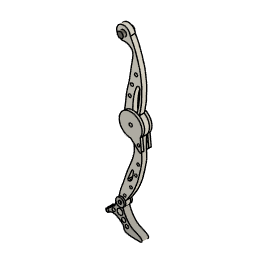
3R Planner Leg (Autodesk Fusion 360 design; units mm, degrees)
Autodesk Fusion 360 part; units mm, degrees
note: some values were not read from the file. Chosen so that the rebuilt part matches the saved one: which face or edge a step refers to. Set by a fixed rule: which sketch regions a step uses.
sketch "Sketch Thigh" plane through (0, 0, 0) normal (0, 1, 0) x (1, 0, 0)
  circle A0 centre (-35.2013, -526.5286) radius 18
  circle A1 centre (-35.2013, -526.5286) radius 42
  circle A2 centre (23.3414, -77.3372) radius 10
  circle A3 centre (23.3414, -77.3372) radius 70
  spline S0 degree 5 poles (-36.4317, -484.5466) (-35.2037, -484.7809) (-32.7765, -485.1866) (-29.2218, -485.606) (-24.6544, -485.7869) (-19.2317, -485.3906) (-14.0932, -484.3977) (-9.2342, -482.86) (-4.6456, -480.8668) (-0.3151, -478.5474) (3.7633, -476.0289) (7.5794, -473.3959) (11.0975, -470.6537) (14.2448, -467.6799) (16.9324, -464.2887) (19.0817, -460.3121) (20.6487, -455.6738) (21.6499, -450.4697) (22.1462, -444.906) (22.2249, -439.2304) (21.9831, -433.6701) (21.5089, -428.3588) (20.8685, -423.2931) (20.1126, -418.3916) (19.2797, -413.5384) (18.4002, -408.6286) (17.5013, -403.6235) (16.6061, -398.5439) (15.7315, -393.4337) (14.8853, -388.3343) (14.0639, -383.2529) (13.2508, -378.1395) (12.4244, -372.9172) (11.5642, -367.5091) (10.6578, -361.8637) (9.7092, -355.9869) (8.7399, -349.9497) (7.778, -343.8514) (6.85, -337.7941) (5.972, -331.8527) (5.1403, -326.0462) (4.323, -320.3093) (3.4714, -314.5275) (2.5311, -308.5697) (1.4536, -302.3234) (0.2063, -295.725) (-1.2135, -288.8021) (-2.7809, -281.6615) (-4.4528, -274.4499) (-6.1756, -267.3234) (-7.8935, -260.4128) (-9.5563, -253.7929) (-11.1279, -247.4427) (-12.5916, -241.2351) (-13.9437, -234.9891) (-15.1909, -228.5075) (-16.3452, -221.6232) (-17.4211, -214.2368) (-18.4302, -206.3689) (-19.3796, -198.1708) (-20.2738, -189.8721) (-21.1157, -181.7419) (-21.908, -174.0454) (-22.6546, -167.0005) (-23.3615, -160.7395) (-24.0388, -155.2553) (-24.7002, -150.407) (-25.3606, -145.9837) (-26.0341, -141.7521) (-26.7323, -137.512) (-27.4617, -133.1445) (-28.073, -129.5011) (-28.5476, -126.6757) (-28.8711, -124.7508) (-29.0347, -123.778) knots 0 0 0 0 0 0 0.01428571 0.02857143 0.04285714 0.05714286 0.07142857 0.08571429 0.1 0.11428571 0.12857143 0.14285714 0.15714286 0.17142857 0.18571429 0.2 0.21428571 0.22857143 0.24285714 0.25714286 0.27142857 0.28571429 0.3 0.31428571 0.32857143 0.34285714 0.35714286 0.37142857 0.38571429 0.4 0.41428571 0.42857143 0.44285714 0.45714286 0.47142857 0.48571429 0.5 0.51428571 0.52857143 0.54285714 0.55714286 0.57142857 0.58571429 0.6 0.61428571 0.62857143 0.64285714 0.65714286 0.67142857 0.68571429 0.7 0.71428571 0.72857143 0.74285714 0.75714286 0.77142857 0.78571429 0.8 0.81428571 0.82857143 0.84285714 0.85714286 0.87142857 0.88571429 0.9 0.91428571 0.92857143 0.94285714 0.95714286 0.97142857 0.98571429 1 1 1 1 1 1
  spline S1 degree 5 poles (6.5737, -530.8697) (7.0819, -529.9673) (8.0856, -528.1802) (9.5529, -525.5529) (11.4329, -522.1561) (13.6572, -518.0832) (15.7611, -514.1707) (17.7553, -510.3927) (19.6573, -506.7066) (21.4946, -503.0462) (23.3012, -499.3289) (25.1103, -495.4746) (26.9465, -491.4225) (28.8195, -487.1472) (30.7152, -482.6796) (32.5963, -478.1064) (34.4167, -473.5372) (36.1326, -469.0815) (37.7154, -464.8201) (39.1618, -460.7812) (40.5096, -456.9081) (41.8236, -453.0843) (43.175, -449.1724) (44.6223, -445.0502) (46.1931, -440.6451) (47.8612, -435.9764) (49.5592, -431.1398) (51.2018, -426.2744) (52.7052, -421.5361) (54.0089, -417.0681) (55.0953, -412.9726) (56.0117, -409.2816) (56.843, -405.9653) (57.681, -402.941) (58.5978, -400.0837) (59.6103, -397.2324) (60.6872, -394.2152) (61.7771, -390.8838) (62.8289, -387.1428) (63.8193, -382.9883) (64.7487, -378.4906) (65.6314, -373.763) (66.4863, -368.9347) (67.3285, -364.1236) (68.1587, -359.4042) (68.9603, -354.7957) (69.7099, -350.2839) (70.3847, -345.8343) (70.971, -341.4096) (71.472, -336.9843) (71.9171, -332.5629) (72.3503, -328.1702) (72.8161, -323.8408) (73.3463, -319.6081) (73.9477, -315.4945) (74.5851, -311.4985) (75.1935, -307.5983) (75.7011, -303.7607) (76.0491, -299.9491) (76.2129, -296.1312) (76.2219, -292.2868) (76.1379, -288.4024) (76.0325, -284.4647) (75.9672, -280.4559) (75.9671, -276.346) (76.0138, -272.0939) (76.0664, -267.6643) (76.0766, -263.0405) (76.0051, -258.2381) (75.8395, -253.3208) (75.6065, -248.4083) (75.3539, -243.6407) (75.136, -239.1482) (74.9971, -235.0179) (74.9579, -231.2653) (74.9959, -227.7929) (75.0547, -224.4212) (75.0665, -220.9505) (74.9679, -217.2076) (74.7222, -213.1105) (74.3246, -208.6794) (73.7907, -203.9948) (73.1489, -199.1682) (72.4317, -194.3094) (71.667, -189.4932) (70.8708, -184.7318) (70.0508, -180.0012) (69.2089, -175.2609) (68.3451, -170.4763) (67.4591, -165.6392) (66.5545, -160.7927) (65.6399, -156.0379) (64.7262, -151.5067) (63.8253, -147.3427) (62.9484, -143.6795) (62.1039, -140.6187) (61.4576, -138.6919) (60.9899, -137.548) (60.6857, -136.9191) (60.5355, -136.6381) knots 0 0 0 0 0 0 0.01052632 0.02105263 0.03157895 0.04210526 0.05263158 0.06315789 0.07368421 0.08421053 0.09473684 0.10526316 0.11578947 0.12631579 0.13684211 0.14736842 0.15789474 0.16842105 0.17894737 0.18947368 0.2 0.21052632 0.22105263 0.23157895 0.24210526 0.25263158 0.26315789 0.27368421 0.28421053 0.29473684 0.30526316 0.31578947 0.32631579 0.33684211 0.34736842 0.35789474 0.36842105 0.37894737 0.38947368 0.4 0.41052632 0.42105263 0.43157895 0.44210526 0.45263158 0.46315789 0.47368421 0.48421053 0.49473684 0.50526316 0.51578947 0.52631579 0.53684211 0.54736842 0.55789474 0.56842105 0.57894737 0.58947368 0.6 0.61052632 0.62105263 0.63157895 0.64210526 0.65263158 0.66315789 0.67368421 0.68421053 0.69473684 0.70526316 0.71578947 0.72631579 0.73684211 0.74736842 0.75789474 0.76842105 0.77894737 0.78947368 0.8 0.81052632 0.82105263 0.83157895 0.84210526 0.85263158 0.86315789 0.87368421 0.88421053 0.89473684 0.90526316 0.91578947 0.92631579 0.93684211 0.94736842 0.95789474 0.96842105 0.97894737 0.98947368 1 1 1 1 1 1
  circle A4 centre (55, -280) radius 9
  circle A5 centre (30, -120) radius 9
  spline S2 degree 5 poles (47.6191, -285.15) (46.8064, -283.5762) (45.2153, -280.4019) (42.9311, -275.5604) (40.0915, -268.9442) (36.8892, -260.4073) (34.038, -251.6146) (31.5388, -242.5934) (29.3866, -233.394) (27.5666, -224.0998) (26.0533, -214.8264) (24.8152, -205.7002) (23.8182, -196.8425) (23.0287, -188.3502) (22.4171, -180.2791) (21.9607, -172.6203) (21.6435, -165.3143) (21.4545, -158.2753) (21.3865, -151.4109) (21.4343, -144.6444) (21.5935, -137.9312) (21.8074, -132.585) (22.0156, -128.5856) (22.1756, -125.9238) (22.2609, -124.5941) knots 0 0 0 0 0 0 0.05 0.1 0.15 0.2 0.25 0.3 0.35 0.4 0.45 0.5 0.55 0.6 0.65 0.7 0.75 0.8 0.85 0.9 0.95 1 1 1 1 1 1
  spline S3 degree 5 poles (63.9903, -280.4171) (63.9954, -279.3418) (63.9944, -277.1207) (63.9589, -273.5771) (63.8437, -268.427) (63.5836, -261.2767) (63.2024, -253.4204) (62.6917, -244.885) (62.0399, -235.7314) (61.2328, -226.0534) (60.2567, -215.9694) (59.1004, -205.6177) (57.7586, -195.15) (56.2338, -184.7277) (54.5407, -174.5163) (52.7057, -164.6805) (50.7617, -155.3773) (48.7441, -146.749) (46.6866, -138.9154) (44.6174, -131.9666) (42.5545, -125.9502) (40.916, -121.8936) (39.695, -119.2752) (38.8845, -117.7173) (38.4801, -116.9853) knots 0 0 0 0 0 0 0.05 0.1 0.15 0.2 0.25 0.3 0.35 0.4 0.45 0.5 0.55 0.6 0.65 0.7 0.75 0.8 0.85 0.9 0.95 1 1 1 1 1 1
  circle A6 centre (41.2295, -343.8614) radius 9
  circle A7 centre (16.4257, -279.8469) radius 9
  circle A8 centre (3.0698, -214.2122) radius 9
  point P0 (-10, -483)
  point P1 (8, -473)
  point P2 (19, -460)
  point P3 (22, -435)
  point P4 (19, -412)
  point P5 (15, -389)
  point P6 (11, -364)
  point P7 (6, -332)
  point P8 (1, -300)
  point P9 (-9, -256)
  point P10 (-17, -217)
  point P11 (-23, -164)
  point P12 (-26, -142)
  point P13 (18.658, -508.6317)
  point P14 (28, -489)
  point P15 (38, -464)
  point P16 (45, -444)
  point P17 (54, -417)
  point P18 (58, -402)
  point P19 (62, -390)
  point P20 (67, -366)
  point P21 (71, -341)
  point P22 (73.5241, -318.4753)
  point P23 (76, -300)
  point P24 (76, -282)
  point P25 (76, -259)
  point P26 (75, -234)
  point P27 (75, -219)
  point P28 (72.5196, -194.9763)
  point P29 (67.7986, -167.5042)
  point P30 (63, -144)
  point P31 (30.2174, -236.7363)
  point P32 (22.9169, -186.5688)
  point P33 (21.4193, -152.687)
  point P34 (63, -250.2474)
  point P35 (56.9337, -189.6784)
  point P36 (45.9709, -136.6381)
  dimension "d1" = 36
  dimension "d2" = 84
  dimension "d3" = 20
  dimension "d4" = 140
  dimension "d5" = 18
  dimension "d6" = 18
  dimension "d7" = 18
  dimension "d8" = 18
  dimension "d9" = 18
  constraint concentric A0 A1
  constraint concentric A2 A3
  constraint coincident A1 S0.start
  constraint coincident A3 S0.end
  constraint coincident A1 S1.start
  constraint coincident A3 S1.end
  constraint coincident A4 S2.start
  constraint coincident A5 S2.end
  constraint coincident A4 S3.start
  constraint coincident A5 S3.end
  measures "d1" diameter of A0
  measures "d2" diameter of A1
  measures "d3" diameter of A2
  measures "d4" diameter of A3
  measures "d5" diameter of A4
  measures "d6" diameter of A5
  measures "d7" diameter of A6
  measures "d8" diameter of A7
  measures "d9" diameter of A8
sketch "Sketch Shin" plane through (0, 0, 0) normal (0, 1, 0) x (1, 0, 0)
  circle A0 centre (23.3414, -77.3372) radius 70
  circle A1 centre (-47.3449, 370.1429) radius 10
  circle A2 centre (-47.3449, 370.1429) radius 26
  line L0 (23.7509, -7.3384) -> (75.8334, 40.3252)
  line L1 (81.648, -38.603) -> (88.8529, 34.857)
  arc A3 (88.8529, 34.857) -> (75.8334, 40.3252) centre (81.4978, 35.5784) ccw
  spline S0 degree 5 poles (-14.5185, -18.4591) (-13.3526, -17.7095) (-10.9184, -16.2466) (-6.9593, -14.1616) (-1.1723, -11.5001) (6.3098, -7.8331) (13.3238, -3.228) (19.226, 2.7745) (23.6918, 10.2286) (26.7608, 18.7607) (28.6795, 27.7924) (29.7939, 36.7053) (30.4327, 45.0106) (30.768, 52.5628) (30.8075, 59.5455) (30.4814, 66.2896) (29.6959, 73.1547) (28.4129, 80.3566) (26.6709, 87.9221) (24.5454, 95.7759) (22.1251, 103.7945) (19.4803, 111.8733) (16.6379, 119.9855) (13.5977, 128.1585) (10.3489, 136.4542) (6.8859, 144.9477) (3.2254, 153.7062) (-0.5796, 162.7696) (-4.4547, 172.1512) (-8.3173, 181.8375) (-12.0912, 191.7877) (-15.7194, 201.9339) (-19.1802, 212.1797) (-22.493, 222.4043) (-25.7012, 232.4817) (-28.8596, 242.2963) (-32.0201, 251.7604) (-35.219, 260.8292) (-38.4607, 269.5218) (-41.7143, 277.9221) (-44.9277, 286.1524) (-48.0377, 294.3529) (-50.9813, 302.661) (-53.707, 311.1873) (-56.1825, 320.0026) (-58.3885, 329.1494) (-59.9305, 336.7481) (-60.9605, 342.6083) (-61.591, 346.5865) (-61.8922, 348.5936) knots 0 0 0 0 0 0 0.022222 0.044444 0.066667 0.088889 0.111111 0.133333 0.155556 0.177778 0.2 0.222222 0.244444 0.266667 0.288889 0.311111 0.333333 0.355556 0.377778 0.4 0.422222 0.444444 0.466667 0.488889 0.511111 0.533333 0.555556 0.577778 0.6 0.622222 0.644444 0.666667 0.688889 0.711111 0.733333 0.755556 0.777778 0.8 0.822222 0.844444 0.866667 0.888889 0.911111 0.933333 0.955556 0.977778 1 1 1 1 1 1
  spline S1 degree 5 poles (75.8334, -31.0275) (75.6679, -27.4473) (75.3638, -20.4187) (74.9879, -10.271) (74.6476, 2.468) (74.4861, 17.0801) (74.5728, 30.4114) (74.8758, 42.5292) (75.3404, 53.552) (75.8833, 63.6625) (76.3864, 73.124) (76.6917, 82.2903) (76.635, 91.5358) (76.0762, 101.19) (74.9297, 111.4729) (73.1985, 122.4227) (70.997, 133.8472) (68.5005, 145.4251) (65.9048, 156.7879) (63.3803, 167.6124) (61.0328, 177.6994) (58.8494, 187.0826) (56.692, 196.042) (54.3645, 204.965) (51.666, 214.2382) (48.4433, 224.1384) (44.6579, 234.696) (40.3986, 245.6719) (35.8234, 256.6886) (31.121, 267.3188) (26.462, 277.1965) (21.9598, 286.1059) (17.6134, 294.113) (13.3307, 301.5063) (8.9894, 308.6463) (4.4849, 315.848) (-0.213, 323.2406) (-5.0177, 330.6622) (-9.7768, 337.7838) (-14.3159, 344.2141) (-18.482, 349.6044) (-21.4523, 352.9381) (-23.465, 354.8632) (-24.7113, 355.891) (-25.3106, 356.341) knots 0 0 0 0 0 0 0.025 0.05 0.075 0.1 0.125 0.15 0.175 0.2 0.225 0.25 0.275 0.3 0.325 0.35 0.375 0.4 0.425 0.45 0.475 0.5 0.525 0.55 0.575 0.6 0.625 0.65 0.675 0.7 0.725 0.75 0.775 0.8 0.825 0.85 0.875 0.9 0.925 0.95 0.975 1 1 1 1 1 1
  spline S2 degree 5 poles (16.717, 171.3852) (15.6483, 173.9298) (13.511, 179.019) (10.3049, 186.6528) (6.0302, 196.8311) (0.6868, 209.5541) (-3.5879, 219.7325) (-6.794, 227.3662) (-8.9313, 232.4554) (-10, 235) knots 0 0 0 0 0 0 0.2 0.4 0.6 0.8 1 1 1 1 1 1
  spline S3 degree 5 poles (-2.8083, 239.0621) (-1.8387, 239.0202) (0.0592, 238.8127) (2.7825, 238.1308) (6.1619, 236.4671) (9.9455, 233.0669) (13.2682, 228.285) (16.1351, 222.1369) (18.5844, 214.7367) (20.6623, 206.2234) (22.4141, 196.7325) (23.5826, 188.4418) (24.3377, 181.86) (24.7881, 177.3132) (25, 175) knots 0 0 0 0 0 0 0.1 0.2 0.3 0.4 0.5 0.6 0.7 0.8 0.9 1 1 1 1 1 1
  circle A4 centre (40, 190) radius 8
  circle A5 centre (10.2637, 267.0264) radius 8
  circle A6 centre (-27.9009, 329.6495) radius 8
  circle A7 centre (53.7528, 125.0461) radius 8
  circle A8 centre (71.5956, 7.1274) radius 8
  circle A9 centre (23.3414, -77.3372) radius 10
  line L2 (-44.533, -37.7591) -> (15.4959, 0.8408)
  arc A10 (16.717, 171.3852) -> (25, 175) centre (20.4005, 174.242) ccw
  arc A11 (-2.8083, 239.0621) -> (-10, 235) centre (-5.3625, 235.1868) ccw
  point P0 (23.3414, -77.3372)
  point P1 (16.1631, 0)
  point P2 (30, 40)
  point P3 (30, 70)
  point P4 (22.1975, 103.3992)
  point P5 (7.1116, 144.3469)
  point P6 (-14.5185, 198.6563)
  point P7 (-33.836, 256.845)
  point P8 (-50, 300)
  point P9 (75.8334, 62.7421)
  point P10 (75, 110)
  point P11 (61.9613, 173.7105)
  point P12 (49.7922, 219.8633)
  point P13 (25, 280)
  point P14 (5, 315)
  point P15 (-15, 345)
  point P16 (11.9184, 229.9613)
  dimension "d10" = 140
  dimension "d11" = 20
  dimension "d12" = 52
  dimension "d13" = 16
  dimension "d14" = 16
  dimension "d15" = 16
  dimension "d16" = 16
  dimension "d17" = 16
  dimension "d18" = 20
  constraint coincident P0 A0.centre
  constraint concentric A1 A2
  constraint coincident A0 L0.start
  constraint coincident A0 L1.start
  constraint tangent L1 A3
  constraint coincident A0 S0.start
  constraint coincident A2 S0.end
  constraint coincident A0 S1.start
  constraint coincident A2 S1.end
  constraint concentric A0 A9
  constraint midpoint S0.start L2
  constraint tangent A0 L2
  measures "d10" diameter of A0
  measures "d11" diameter of A1
  measures "d12" diameter of A2
  measures "d13" diameter of A4
  measures "d14" diameter of A5
  measures "d15" diameter of A6
  measures "d16" diameter of A7
  measures "d17" diameter of A8
  measures "d18" diameter of A9
sketch "Sketch Foot" plane through (0, 0, 0) normal (0, 1, 0) x (1, 0, 0)
  circle A0 centre (-47.3449, 370.1429) radius 10
  circle A1 centre (-47.3449, 370.1429) radius 26
  circle A2 centre (-128.2734, 454.5835) radius 11
  circle A3 centre (-128.2734, 454.5835) radius 8
  circle A4 centre (-90.61, 433.3591) radius 10
  circle A5 centre (-52.2357, 425.8836) radius 17
  circle A6 centre (-29.8093, 456.9484) radius 12.5
  circle A7 centre (-10.2068, 482.3651) radius 10
  spline S0 degree 5 poles (-69.8612, 357.1424) (-70.3793, 358.0322) (-71.3687, 359.8879) (-72.7128, 362.8993) (-74.223, 367.3734) (-75.6696, 373.6933) (-76.7588, 380.6291) (-77.6942, 387.9053) (-78.7713, 395.1215) (-80.5825, 401.4685) (-83.3469, 406.6564) (-86.9553, 410.8441) (-91.1343, 414.4058) (-95.5458, 417.7867) (-99.924, 421.3045) (-104.1598, 425.0282) (-108.2458, 428.8711) (-112.242, 432.6498) (-116.2374, 436.1505) (-120.3099, 439.2002) (-124.5011, 441.7082) (-127.9653, 443.2483) (-130.6284, 444.1375) (-132.4325, 444.6126) (-133.3417, 444.8207) knots 0 0 0 0 0 0 0.05 0.1 0.15 0.2 0.25 0.3 0.35 0.4 0.45 0.5 0.55 0.6 0.65 0.7 0.75 0.8 0.85 0.9 0.95 1 1 1 1 1 1
  spline S1 degree 5 poles (-119.4476, 461.149) (-119.1432, 460.6511) (-118.4608, 459.6828) (-117.2168, 458.3124) (-115.1171, 456.6497) (-111.7803, 454.8532) (-107.7983, 453.3614) (-103.3125, 452.2212) (-98.5123, 451.4925) (-93.5938, 451.2305) (-88.7268, 451.4718) (-84.0103, 452.215) (-79.4604, 453.4163) (-75.05, 455.0081) (-70.7362, 456.9121) (-66.4922, 459.0547) (-62.3394, 461.3821) (-58.3255, 463.8558) (-54.4954, 466.4457) (-50.8694, 469.1254) (-47.407, 471.864) (-44.0231, 474.6308) (-40.6602, 477.4174) (-37.336, 480.251) (-34.2231, 483.2186) (-31.6413, 486.462) (-29.8557, 490.107) (-28.9381, 494.2136) (-28.553, 498.7015) (-27.9609, 503.3469) (-26.2855, 507.8633) (-22.7119, 511.9618) (-16.717, 515.4203) (-8.2752, 518.146) (2.2562, 520.1455) (14.2417, 521.4986) (26.8756, 522.3306) (39.2873, 522.7855) (50.6504, 522.9982) (60.2843, 523.0684) (67.771, 523.031) (73.0402, 522.8348) (76.5326, 522.2998) (78.9409, 521.1898) (80.8652, 519.31) (82.4013, 516.6194) (83.0845, 513.2569) (82.3173, 509.4455) (79.7439, 505.4159) (75.4161, 501.3583) (69.6293, 497.4276) (62.8484, 493.7338) (55.5942, 490.3375) (48.3546, 487.2454) (41.4662, 484.4015) (35.08, 481.6938) (29.2192, 478.9773) (23.8128, 476.0936) (18.7391, 472.8912) (13.8632, 469.2453) (9.0815, 465.0797) (4.3512, 460.3812) (-0.327, 455.1822) (-4.9178, 449.5496) (-9.3644, 443.5712) (-13.5996, 437.3427) (-17.5566, 430.9552) (-21.1831, 424.4808) (-24.4425, 417.9697) (-27.3107, 411.4559) (-29.7736, 404.9595) (-31.4144, 399.7844) (-32.4586, 395.9169) (-33.0721, 393.3448) (-33.3581, 392.0602) knots 0 0 0 0 0 0 0.01428571 0.02857143 0.04285714 0.05714286 0.07142857 0.08571429 0.1 0.11428571 0.12857143 0.14285714 0.15714286 0.17142857 0.18571429 0.2 0.21428571 0.22857143 0.24285714 0.25714286 0.27142857 0.28571429 0.3 0.31428571 0.32857143 0.34285714 0.35714286 0.37142857 0.38571429 0.4 0.41428571 0.42857143 0.44285714 0.45714286 0.47142857 0.48571429 0.5 0.51428571 0.52857143 0.54285714 0.55714286 0.57142857 0.58571429 0.6 0.61428571 0.62857143 0.64285714 0.65714286 0.67142857 0.68571429 0.7 0.71428571 0.72857143 0.74285714 0.75714286 0.77142857 0.78571429 0.8 0.81428571 0.82857143 0.84285714 0.85714286 0.87142857 0.88571429 0.9 0.91428571 0.92857143 0.94285714 0.95714286 0.97142857 0.98571429 1 1 1 1 1 1
  line L0 (-75.8888, 378.6486) -> (-81.1768, 407.0206)
  point P0 (-47.3449, 370.1429)
  point P1 (-78.5328, 392.8346)
  point P2 (-94.5259, 417.0193)
  point P3 (-115, 435)
  point P4 (-110.8193, 454.5835)
  point P5 (-90.61, 451.4454)
  point P6 (-70.4641, 457.1093)
  point P7 (-52.7191, 467.7848)
  point P8 (-38.4765, 479.3144)
  point P9 (-29.4337, 492.4266)
  point P10 (-22.3124, 511.6427)
  point P11 (68.7733, 522.9521)
  point P12 (80, 520)
  point P13 (82.461, 511.1523)
  point P14 (51.7816, 488.7327)
  point P15 (15, 470)
  point P16 (-15, 435)
  dimension "d19" = 20
  dimension "d20" = 52
  dimension "d21" = 22
  dimension "d22" = 16
  dimension "d23" = 20
  dimension "d24" = 34
  dimension "d25" = 25
  dimension "d26" = 20
  constraint coincident P0 A0.centre
  constraint concentric A2 A3
  constraint coincident A1 S0.start
  constraint coincident A2 S0.end
  constraint coincident A1 S1.end
  constraint coincident A2 S1.start
  constraint midpoint P1 L0
  measures "d19" diameter of A0
  measures "d20" diameter of A1
  measures "d21" diameter of A2
  measures "d22" diameter of A3
  measures "d23" diameter of A4
  measures "d24" diameter of A5
  measures "d25" diameter of A6
  measures "d26" diameter of A7
extrude "Extrude1" add sketch "Sketch Thigh" along normal mid plane 30 contours A1 S0 | A1 A3 S0 S1 A4 S2 S3 | A3 A5 S2 S3 picked at (-24.6319, -494.3073) picked at (2.825, -108.3208) makes body 1
extrude "Extrude2" add sketch "Sketch Shin" along normal mid plane 30 separate body contours A0 L0 S1 A8 | A0 A2 L0 S0 S1 | S1 A8 | A2 picked at (68.2154, 5.7087) makes body 2
extrude "Extrude3" add sketch "Sketch Shin" along normal blind 15 from surface at 15 contours A0 S0 | A0 L0 L1 A3 S1 A8 | A0 S0 | A0 L0 S1 A8 bodies 2
extrude "Extrude4" add sketch "Sketch Shin" against normal blind 15 from surface at -15 contours A0 S0 | A0 L0 L1 A3 S1 A8 | A0 S0 | A0 L0 S1 A8 bodies 2
extrude "Extrude5" add sketch "Sketch Foot" along normal mid plane 40 separate body contours A1 A2 S0 S1 | A2 S0 S1 makes body 3
extrude "Extrude6" add sketch "Sketch Foot" along normal blind 10 from surface at 15 contours A1 bodies 3
extrude "Extrude7" add sketch "Sketch Foot" against normal blind 10 from surface at -15 contours A1 bodies 3
sketch "Sketch4" plane through (0, -15, 0) normal (0, -1, 0) x (1, 0, 0)
  arc A0 (63.9928, 279.6408) -> (46.4872, 282.9211) centre (55, 280) ccw
  spline S0 degree 5 poles (63.9928, 279.6408) (63.9944, 278.702) (63.9889, 276.6116) (63.9505, 273.208) (63.8362, 268.2225) (63.5836, 261.2767) (63.2024, 253.4204) (62.6917, 244.885) (62.0399, 235.7314) (61.2328, 226.0534) (60.2567, 215.9694) (59.1004, 205.6177) (57.7586, 195.15) (56.2338, 184.7277) (54.5407, 174.5163) (52.7057, 164.6805) (50.7617, 155.3773) (48.7441, 146.749) (46.6866, 138.9154) (44.6174, 131.9666) (42.5545, 125.9502) (40.916, 121.8936) (39.695, 119.2752) (38.8845, 117.7173) (38.4801, 116.9853) knots 0.007153 0.007153 0.007153 0.007153 0.007153 0.007153 0.05 0.1 0.15 0.2 0.25 0.3 0.35 0.4 0.45 0.5 0.55 0.6 0.65 0.7 0.75 0.8 0.85 0.9 0.95 1 1 1 1 1 1
  arc A1 (22.2609, 124.5941) -> (38.4801, 116.9853) centre (30, 120) ccw
  spline S1 degree 5 poles (22.2609, 124.5941) (22.1756, 125.9238) (22.0156, 128.5856) (21.8074, 132.585) (21.5935, 137.9312) (21.4343, 144.6444) (21.3865, 151.4109) (21.4545, 158.2753) (21.6435, 165.3143) (21.9607, 172.6203) (22.4171, 180.2791) (23.0287, 188.3502) (23.8182, 196.8425) (24.8152, 205.7002) (26.0533, 214.8264) (27.5666, 224.0998) (29.3866, 233.394) (31.5388, 242.5934) (34.038, 251.6146) (36.8892, 260.4073) (39.9109, 268.4628) (42.5322, 274.6267) (44.5755, 279.0338) (45.9175, 281.7801) (46.4872, 282.9211) knots -1 -1 -1 -1 -1 -1 -0.95 -0.9 -0.85 -0.8 -0.75 -0.7 -0.65 -0.6 -0.55 -0.5 -0.45 -0.4 -0.35 -0.3 -0.25 -0.2 -0.15 -0.1 -0.05 -0.014095 -0.014095 -0.014095 -0.014095 -0.014095 -0.014095
  circle A2 centre (41.2295, 343.8614) radius 9
  circle A3 centre (16.4257, 279.8469) radius 9
  circle A4 centre (-35.2013, 526.5286) radius 18
  circle A5 centre (3.0698, 214.2122) radius 9
  circle A6 centre (23.3414, 77.3372) radius 10
  arc A7 (6.5737, 530.8697) -> (-36.4317, 484.5466) centre (-35.2013, 526.5286) ccw
  spline S2 degree 5 poles (-36.4317, 484.5466) (-35.2037, 484.7809) (-32.9698, 485.1543) (-30.7846, 485.4209) (-28.6479, 485.5806) (-26.5599, 485.6344) (-25.6163, 485.6369) knots 0 0 0 0 0 0 0.014286 0.026296 0.026296 0.026296 0.026296 0.026296 0.026296
  spline S3 degree 5 poles (-25.6163, 485.6369) (-25.4375, 485.6374) (-24.139, 485.6352) (-21.7563, 485.5533) (-18.3677, 485.2236) (-14.0932, 484.3977) (-9.2342, 482.86) (-4.6456, 480.8668) (-0.3151, 478.5474) (3.7633, 476.0289) (7.5794, 473.3959) (11.0975, 470.6537) (14.2448, 467.6799) (16.9324, 464.2887) (19.0817, 460.3121) (20.6487, 455.6738) (21.6499, 450.4697) (22.1462, 444.906) (22.2249, 439.2304) (21.9831, 433.6701) (21.5089, 428.3588) (20.8685, 423.2931) (20.1126, 418.3916) (19.2797, 413.5384) (18.4002, 408.6286) (17.5013, 403.6235) (16.6061, 398.5439) (15.7315, 393.4337) (14.8853, 388.3343) (14.0639, 383.2529) (13.2508, 378.1395) (12.4244, 372.9172) (11.5642, 367.5091) (10.6578, 361.8637) (9.7092, 355.9869) (8.7399, 349.9497) (7.778, 343.8514) (6.85, 337.7941) (5.972, 331.8527) (5.1403, 326.0462) (4.323, 320.3093) (3.4714, 314.5275) (2.5311, 308.5697) (1.4536, 302.3234) (0.2063, 295.725) (-1.2135, 288.8021) (-2.7809, 281.6615) (-4.4528, 274.4499) (-6.1756, 267.3234) (-7.8935, 260.4128) (-9.5563, 253.7929) (-11.1279, 247.4427) (-12.5916, 241.2351) (-13.9437, 234.9891) (-15.1909, 228.5075) (-16.3452, 221.6232) (-17.4211, 214.2368) (-18.4302, 206.3689) (-19.3796, 198.1708) (-20.2738, 189.8721) (-21.1157, 181.7419) (-21.908, 174.0454) (-22.6546, 167.0005) (-23.3615, 160.7395) (-24.0388, 155.2553) (-24.7002, 150.407) (-25.3606, 145.9837) (-26.0341, 141.7521) (-26.7323, 137.512) (-27.4617, 133.1445) (-28.073, 129.5011) (-28.5476, 126.6757) (-28.8711, 124.7508) (-29.0347, 123.778) knots 0.02629564 0.02629564 0.02629564 0.02629564 0.02629564 0.02629564 0.02857143 0.04285714 0.05714286 0.07142857 0.08571429 0.1 0.11428571 0.12857143 0.14285714 0.15714286 0.17142857 0.18571429 0.2 0.21428571 0.22857143 0.24285714 0.25714286 0.27142857 0.28571429 0.3 0.31428571 0.32857143 0.34285714 0.35714286 0.37142857 0.38571429 0.4 0.41428571 0.42857143 0.44285714 0.45714286 0.47142857 0.48571429 0.5 0.51428571 0.52857143 0.54285714 0.55714286 0.57142857 0.58571429 0.6 0.61428571 0.62857143 0.64285714 0.65714286 0.67142857 0.68571429 0.7 0.71428571 0.72857143 0.74285714 0.75714286 0.77142857 0.78571429 0.8 0.81428571 0.82857143 0.84285714 0.85714286 0.87142857 0.88571429 0.9 0.91428571 0.92857143 0.94285714 0.95714286 0.97142857 0.98571429 1 1 1 1 1 1
  arc A8 (-29.0347, 123.778) -> (60.5355, 136.6381) centre (23.3414, 77.3372) ccw
  spline S4 degree 5 poles (60.5355, 136.6381) (60.6857, 136.9191) (60.9899, 137.548) (61.4576, 138.6919) (62.1039, 140.6187) (62.9484, 143.6795) (63.8253, 147.3427) (64.7262, 151.5067) (65.6399, 156.0379) (66.5545, 160.7927) (67.4591, 165.6392) (68.3451, 170.4763) (69.2089, 175.2609) (70.0508, 180.0012) (70.8708, 184.7318) (71.667, 189.4932) (72.4317, 194.3094) (73.1489, 199.1682) (73.7907, 203.9948) (74.3246, 208.6794) (74.7222, 213.1105) (74.9679, 217.2076) (75.0665, 220.9505) (75.0547, 224.4212) (74.9959, 227.7929) (74.9579, 231.2653) (74.9971, 235.0179) (75.136, 239.1482) (75.3539, 243.6407) (75.6065, 248.4083) (75.8395, 253.3208) (76.0051, 258.2381) (76.0766, 263.0405) (76.0664, 267.6643) (76.0138, 272.0939) (75.9671, 276.346) (75.9672, 280.4559) (76.0325, 284.4647) (76.1379, 288.4024) (76.2219, 292.2868) (76.2129, 296.1312) (76.0491, 299.9491) (75.7011, 303.7607) (75.1935, 307.5983) (74.5851, 311.4985) (73.9477, 315.4945) (73.3463, 319.6081) (72.8161, 323.8408) (72.3503, 328.1702) (71.9171, 332.5629) (71.472, 336.9843) (70.971, 341.4096) (70.3847, 345.8343) (69.7099, 350.2839) (68.9603, 354.7957) (68.1587, 359.4042) (67.3285, 364.1236) (66.4863, 368.9347) (65.6314, 373.763) (64.7487, 378.4906) (63.8193, 382.9883) (62.8289, 387.1428) (61.7771, 390.8838) (60.6872, 394.2152) (59.6103, 397.2324) (58.5978, 400.0837) (57.681, 402.941) (56.843, 405.9653) (56.0117, 409.2816) (55.0953, 412.9726) (54.0089, 417.0681) (52.7052, 421.5361) (51.2018, 426.2744) (49.5592, 431.1398) (47.8612, 435.9764) (46.1931, 440.6451) (44.6223, 445.0502) (43.175, 449.1724) (41.8236, 453.0843) (40.5096, 456.9081) (39.1618, 460.7812) (37.7154, 464.8201) (36.1326, 469.0815) (34.4167, 473.5372) (32.5963, 478.1064) (30.7152, 482.6796) (28.8195, 487.1472) (26.9465, 491.4225) (25.1103, 495.4746) (23.3012, 499.3289) (21.4946, 503.0462) (19.6573, 506.7066) (17.7553, 510.3927) (15.7611, 514.1707) (13.6572, 518.0832) (11.4329, 522.1561) (9.5529, 525.5529) (8.0856, 528.1802) (7.0819, 529.9673) (6.5737, 530.8697) knots -1 -1 -1 -1 -1 -1 -0.98947368 -0.97894737 -0.96842105 -0.95789474 -0.94736842 -0.93684211 -0.92631579 -0.91578947 -0.90526316 -0.89473684 -0.88421053 -0.87368421 -0.86315789 -0.85263158 -0.84210526 -0.83157895 -0.82105263 -0.81052632 -0.8 -0.78947368 -0.77894737 -0.76842105 -0.75789474 -0.74736842 -0.73684211 -0.72631579 -0.71578947 -0.70526316 -0.69473684 -0.68421053 -0.67368421 -0.66315789 -0.65263158 -0.64210526 -0.63157895 -0.62105263 -0.61052632 -0.6 -0.58947368 -0.57894737 -0.56842105 -0.55789474 -0.54736842 -0.53684211 -0.52631579 -0.51578947 -0.50526316 -0.49473684 -0.48421053 -0.47368421 -0.46315789 -0.45263158 -0.44210526 -0.43157895 -0.42105263 -0.41052632 -0.4 -0.38947368 -0.37894737 -0.36842105 -0.35789474 -0.34736842 -0.33684211 -0.32631579 -0.31578947 -0.30526316 -0.29473684 -0.28421053 -0.27368421 -0.26315789 -0.25263158 -0.24210526 -0.23157895 -0.22105263 -0.21052632 -0.2 -0.18947368 -0.17894737 -0.16842105 -0.15789474 -0.14736842 -0.13684211 -0.12631579 -0.11578947 -0.10526316 -0.09473684 -0.08421053 -0.07368421 -0.06315789 -0.05263158 -0.04210526 -0.03157895 -0.02105263 -0.01052632 0 0 0 0 0 0
  circle A9 centre (-35.2013, 526.5286) radius 18
  constraint concentric A4 A9
extrude "Extrude8" add sketch "Sketch4" along normal blind 20 and the other way blind 50 separate body contours A4 A9 makes body 4
copy_body "Body->Comp1" bodies 1 removing the originals makes body 5 in component "Thigh"
copy_body "Body->Comp2" bodies 2 removing the originals makes body 6 in component "Shin"
copy_body "Body->Comp3" bodies 3 removing the originals makes body 7 in component "Foot"
copy_body "Body->Comp4" bodies 4 removing the originals makes body 8 in component "Shaft"
component "Shin" placed x (1, 0, 0) y (0, 1, 0) z (0, 0, 1) at (0, 0, 0)
component "Foot" placed x (1, 0, 0) y (0, 1, 0) z (0, 0, 1) at (0, 0, 0)
component "Shaft" placed x (1, 0, 0) y (0, 1, 0) z (0, 0, 1) at (0, 0, 0)
component "Thigh" placed x (1, 0, 0) y (0, 1, 0) z (0, 0, 1) at (0, 0, 0)
